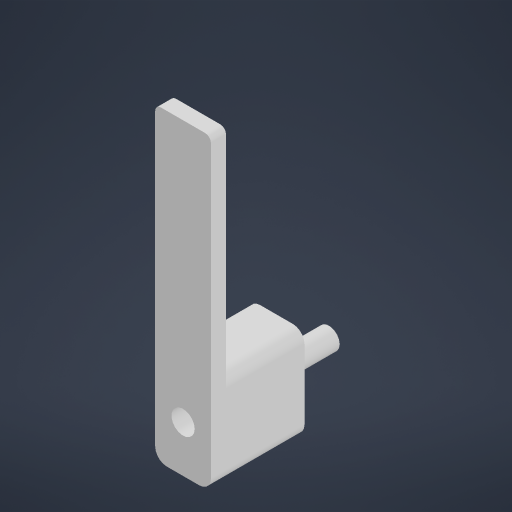
# Autodesk Inventor part: Hook_TestFit
Saved by Autodesk Inventor 2024.1 (Build 281209000, 209)
## iProperties
Created: 2023-07-11
Part Number: Hook_TestFit
Material: Generic
Document SubType Name: Modeling
Designer: User
Density: 1 g/cm^3
Appearance: Default
Author: User
Autodesk Inventor part; units mm, degrees
ref_plane "YZ Plane" through (0, 0, 0) normal (1, 0, 0) x (0, 1, 0)
ref_plane "XZ Plane" through (0, 0, 0) normal (0, 1, 0) x (-1, 0, 0)
ref_plane "XY Plane" through (0, 0, 0) normal (0, 0, 1) x (1, 0, 0)
sketch "Sketch8" plane through (0, 0, 0) normal (0, 0, 1) x (1, 0, 0)
  line L0 (0, 0) -> (-9.6, 0)
  line L1 (-9.6, 0) -> (-9.6, 53)
  line L2 (-9.6, 53) -> (0, 53)
  line L3 (0, 53) -> (0, 0)
  line L4 (0, 4) -> (-9.6, 4)
  line L5 (-4.8, 4) -> (-4.8, 12)
  circle A0 centre (-4.8, 8) radius 2
  point P0 (-4.8, 6)
  point P1 (-4.8, 10)
  dimension "d23" = 9.6
  dimension "d24" = 53
  dimension "d25" = 8
  dimension "d26" = 4
  constraints: 12 end point, 4 point on line, 2 midpoint, 2 parallel, 2 perpendicular, 1 centre point, 1 horizontal, 1 vertical
  measures "d23" distance of L1.end L2.end
  measures "d24" distance of L0.end L1.end
  measures "d25" distance of L5.start L5.end
  measures "d26" diameter of A0
extrude "Extrusion7" add sketch "Sketch8" along normal blind 2.6
sketch "Sketch9" plane through (0, 0, 0) normal (0, 0, -1) x (-1, 0, 0)
  line L0 (0, 0) -> (9.6, 0)
  line L1 (9.6, 0) -> (9.6, 16)
  line L2 (9.6, 16) -> (0, 16)
  line L3 (0, 16) -> (0, 0)
  dimension "d29" = 9.6
  dimension "d30" = 16
  constraints: 8 end point, 2 parallel, 1 horizontal, 1 perpendicular
  measures "d29" distance of L2.end L1.end
  measures "d30" distance of L1.end L0.end
extrude "Extrusion8" add sketch "Sketch9" along normal blind 13.5
sketch "Sketch10" plane through (0, 0, -13.5) normal (0, 0, -1) x (-1, 0, 0)
  circle A0 centre (4.8, 8) radius 1.75
  circle A1 centre (4.8, 8) radius 1.85
  point P0 (0, 0)
  dimension "d33" = 3.5
  dimension "d41" = 3.7
  constraints: 2 centre point, 1 coincident
  measures "d33" diameter of A0
  measures "d41" diameter of A1
extrude "Extrusion9" add sketch "Sketch10" along normal blind 9 contours A0 | A1
fillet "Fillet2" radius 2 4 edges at (-9.6, 16, -6.75) (0, 16, -6.75) (-9.6, 0, -5.45) (0, 0, -5.45)
fillet "Fillet3" radius 1 2 edges at (-9.6, 53, 1.3) (0, 53, 1.3)
sketch "Sketch11" plane through (-4.8, 8, 0) normal (0, 0, 1) x (1, 0, 0)
  circle A0 centre (0, 0) radius 2
  point P0 (4.8, -8)
  dimension "d38" = 4
  constraints: 1 centre point
  measures "d38" diameter of A0
extrude "Extrusion10" cut sketch "Sketch11" against normal blind 10
body "Solid2"
